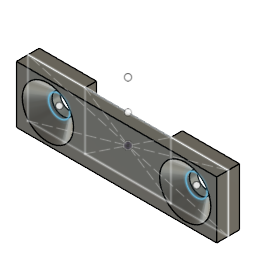
cable management (Autodesk Fusion 360 design; units mm, degrees)
Autodesk Fusion 360 part; units mm, degrees
sketch "Sketch1" plane through (0, 0, 0) normal (0, 1, 0) x (1, 0, 0)
  line L0 (-17.5, 5) -> (17.5, 5)
  line L1 (17.5, 5) -> (17.5, -5)
  line L2 (17.5, -5) -> (-17.5, -5)
  line L3 (-17.5, -5) -> (-17.5, 5)
  line L4 (-17.5, 5) -> (17.5, -5) construction
  line L5 (17.5, 5) -> (-17.5, -5) construction
  line L6 (-7.5, 5) -> (7.5, 5)
  line L7 (7.5, 5) -> (7.5, -5)
  line L8 (7.5, -5) -> (-7.5, -5)
  line L9 (-7.5, -5) -> (-7.5, 5)
  line L10 (-7.5, 5) -> (7.5, -5) construction
  line L11 (7.5, 5) -> (-7.5, -5) construction
  circle A0 centre (-12, 0) radius 1.875
  line L12 (0, -5) -> (0, -10.3309) construction
  line L13 (0, -5) -> (0, -10.3309) construction
  circle A1 centre (12, 0) radius 1.875
  dimension "d1" = 15
  dimension "d2" = 35
  dimension "d3" = 10
  dimension "d4" = 3.75
  constraint horizontal L0
  constraint perpendicular L0 L1
  constraint parallel L0 L2
  constraint parallel L1 L3
  constraint coincident L4 origin
  constraint coincident L5 origin
  constraint horizontal L6
  constraint perpendicular L6 L7
  constraint parallel L6 L8
  constraint parallel L7 L9
  constraint coincident L10 origin
  constraint coincident L11 origin
  constraint coincident L0 L6.start
  constraint midpoint L8 L12.start
  constraint perpendicular L2 L12
  constraint symmetric A0 L12 A1
  constraint symmetric L13.start L12 L12.start
  constraint symmetric L13.end L12 L12.end
  measures "d1" distance of L7 L9
  measures "d2" distance of L0.start L0.end
  measures "d3" distance of L0.end L1.end
  measures "d4" diameter of A0
extrude "Extrude1" add sketch "Sketch1" along normal blind 2 contours L0 L2 L3 L9 | L0 L1 L2 L7 makes body 1 at (-16.2917, 0, 0) makes body 2 at (16.2917, 0, 0)
extrude "Extrude2" add sketch "Sketch1" against normal blind 2 bodies 1 2
chamfer "Chamfer1" distance 2.6 angle 45 2 edges at (-13.7481, -2, 0.678) (10.2519, -2, 0.678) on bodies 1
equation "d2 = 15 mm + 4 mm + 4 mm + 8 mm + 4 mm"
